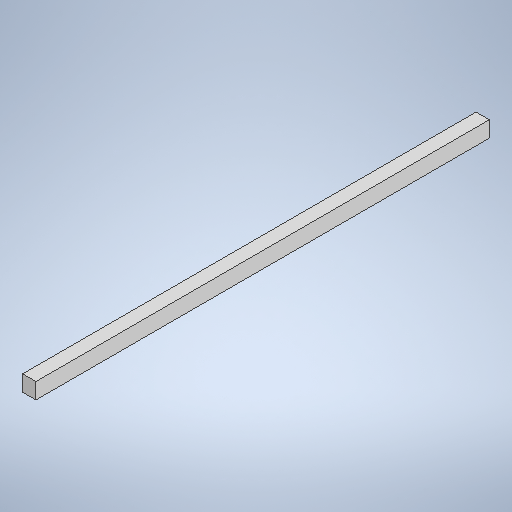
# Autodesk Inventor part: scrambler_spider_support2
Saved by Autodesk Inventor 2025.2 (Build 292293000, 293)
## iProperties
Created: 2025-10-14
Part Number: scrambler_spider_support2
Material: Generic
Document SubType Name: Modeling
Designer: pascu
Density: 1 g/cm^3
Appearance: Default
Author: pascu
Autodesk Inventor part; units mm, degrees
ref_plane "YZ Plane" through (0, 0, 0) normal (1, 0, 0) x (0, 1, 0)
ref_plane "XZ Plane" through (0, 0, 0) normal (0, 1, 0) x (-1, 0, 0)
ref_plane "XY Plane" through (0, 0, 0) normal (0, 0, 1) x (1, 0, 0)
sketch "Sketch1" plane through (0, 0, 0) normal (0, 1, 0) x (-1, 0, 0)
  line L0 (0, 0) -> (-3.175, 0)
  line L1 (-3.175, 0) -> (-3.175, -108.2294)
  line L2 (-3.175, -108.2294) -> (0, -108.2294)
  line L3 (0, -108.2294) -> (0, 0)
  dimension "d0" = 3.175
  dimension "d1" = 108.2294
  constraints: 8 end point, 2 parallel, 1 horizontal, 1 perpendicular
  measures "d0" distance of L2.end L1.end
  measures "d1" distance of L1.end L0.end
extrude "Extrusion1" add sketch "Sketch1" along normal blind 3.81
body "Solid1"
